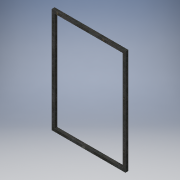
# Autodesk Inventor part: Steel support 5
Saved by Autodesk Inventor 2019 (Build 230136000, 136)
## iProperties
Created: 2021-03-08
Part Number: Steel support 5
Material: Steel
Document SubType Name: Modeling
Designer: User
Density: 7.85 g/cm^3
Appearance: Plate
Author: User
Autodesk Inventor part; units mm, degrees
ref_plane "YZ Plane" through (0, 0, 0) normal (1, 0, 0) x (0, 1, 0)
ref_plane "XZ Plane" through (0, 0, 0) normal (0, 1, 0) x (-1, 0, 0)
ref_plane "XY Plane" through (0, 0, 0) normal (0, 0, 1) x (1, 0, 0)
sketch "Sketch1" plane through (0, 0, 0) normal (0, 0, 1) x (1, 0, 0)
  line L0 (-129.2308, 249.2308) -> (150.7692, 249.2308)
  line L1 (150.7692, 249.2308) -> (150.7692, -150.7692)
  line L2 (150.7692, -150.7692) -> (-129.2308, -150.7692)
  line L3 (-129.2308, -150.7692) -> (-129.2308, 249.2308)
  line L4 (-119.2308, 239.2308) -> (140.7692, 239.2308)
  line L5 (140.7692, 239.2308) -> (140.7692, -140.7692)
  line L6 (140.7692, -140.7692) -> (-119.2308, -140.7692)
  line L7 (-119.2308, -140.7692) -> (-119.2308, 239.2308)
  point P0 (0, 0)
  dimension "d0" = 280
  dimension "d1" = 400
  dimension "d2" = 10
  dimension "d3" = 10
  dimension "d4" = 10
  dimension "d5" = 10
  dimension "d6" = 150.7692
  dimension "d7" = 249.2308
  constraints: 16 end point, 4 parallel, 2 horizontal, 2 perpendicular
  measures "d0" distance between parallel lines of L1 L3
  measures "d1" distance between parallel lines of L0 L2
  measures "d2" distance between parallel lines of L0 L4
  measures "d3" distance between parallel lines of L2 L6
  measures "d4" distance between parallel lines of L1 L5
  measures "d5" distance between parallel lines of L3 L7
  measures "d6" distance from line of point (0, 0) L1
  measures "d7" distance from line of point (0, 0) L0
extrude "Extrusion1" add sketch "Sketch1" along normal mid plane 10
body "Solid1"
